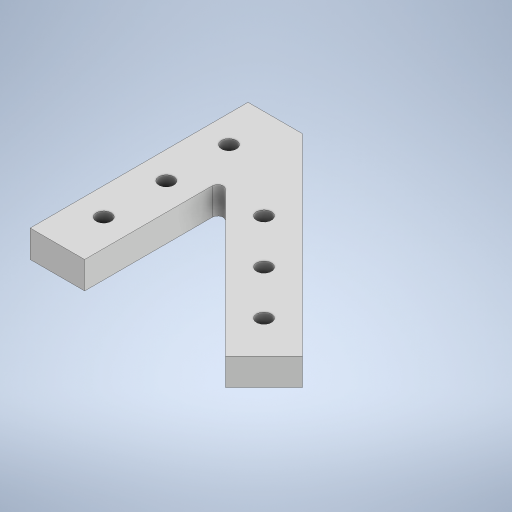
# Autodesk Inventor part: Back_Hip_Bracket
Saved by Autodesk Inventor 2023 (Build 270158000, 158)
## iProperties
Created: 2023-02-16
Part Number: Back_Hip_Bracket
Material: Generic
Document SubType Name: Modeling
Designer: bugme
Density: 1 g/cm^3
Appearance: Default
Author: bugme
Autodesk Inventor part; units mm, degrees
ref_plane "YZ Plane" through (0, 0, 0) normal (1, 0, 0) x (0, 1, 0)
ref_plane "XZ Plane" through (0, 0, 0) normal (0, 1, 0) x (-1, 0, 0)
ref_plane "XY Plane" through (0, 0, 0) normal (0, 0, 1) x (1, 0, 0)
sketch "Sketch2" plane through (0, 0, 0) normal (0, 1, 0) x (-1, 0, 0)
  line L0 (0, 28.2843) -> (-56.5685, 84.8528)
  line L1 (-56.5685, 84.8528) -> (-70.7107, 70.7107)
  line L2 (-70.7107, 70.7107) -> (0, 0)
  line L3 (0, 0) -> (20, 0)
  line L4 (20, 0) -> (20, 80)
  line L5 (20, 80) -> (0, 80)
  line L6 (0, 28.2843) -> (0, 80)
  circle A0 centre (10, 63) radius 2.7559
  circle A1 centre (10, 40) radius 2.7559
  circle A2 centre (10, 17) radius 2.7559
  circle A3 centre (-51.6188, 65.7609) radius 2.7559
  circle A4 centre (-35.3553, 49.4975) radius 2.7559
  circle A5 centre (-19.0919, 33.234) radius 2.7559
  dimension "d10" = 20
  dimension "d11" = 100
  dimension "d12" = 45
  dimension "d13" = 51.7157
  dimension "d15" = 135
  dimension "d16" = 5.5118
  dimension "d20" = 23
  dimension "d28" = 23
  dimension "d33" = 80
  dimension "d34" = 10
  dimension "d35" = 17
  dimension "d36" = 10
  dimension "d37" = 17
  constraints: 14 end point, 6 centre point, 3 equal length, 2 parallel, 1 equal radius, 1 horizontal, 1 vertical, 9 other
  measures "d10" distance of L2.end L3.end
  measures "d11" distance of L1.end L2.end
  measures "d12" angle of L0 L6
  measures "d13" distance of L0.start L5.end
  measures "d15" angle of L2 L3
  measures "d16" diameter of A0
  measures "d20" distance of A0.centre A1.centre
  measures "d28" distance of A3.centre A4.centre
  measures "d33" distance of L0.start L0.end
  measures "d34" distance from line of L6 A0.centre
  measures "d35" distance from line of L5 A0.centre
  measures "d36" distance from line of L2 A3.centre
  measures "d37" distance from line of L1 A3.centre
extrude "Extrusion1" add sketch "Sketch2" along normal blind 10
fillet "Fillet1" radius 2 1 edges at (0, 5, 28.2843)
equation "\"d13\" = d33 - d14"
equation "\"d20\" = -d35 + 0.5 * d33"
equation "\"d28\" = d20"
equation "\"d36\" = d34"
equation "\"d37\" = d35"
equation "\"d14\" = 28.284271"
body "Solid1"
